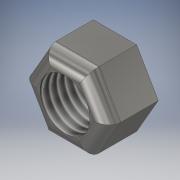
# Autodesk Inventor part: LucasCharles part 5 nut final
Saved by Autodesk Inventor 2018 (Build 220112000, 112)
## iProperties
Created: 2018-05-16
Part Number: LucasCharles part 5 nut final
Material: Stainless Steel, Austenitic
Document SubType Name: Modeling
Designer: 21lsilva
Density: 8 g/cm^3
Appearance: Semi-Polished
Author: 21lsilva
Autodesk Inventor part; units mm, degrees
ref_plane "YZ Plane" through (0, 0, 0) normal (1, 0, 0) x (0, 1, 0)
ref_plane "XZ Plane" through (0, 0, 0) normal (0, 1, 0) x (-1, 0, 0)
ref_plane "XY Plane" through (0, 0, 0) normal (0, 0, 1) x (1, 0, 0)
sketch "Sketch1" plane through (0, 0, 0) normal (0, 0, 1) x (1, 0, 0)
  line L0 (-10.9985, 0) -> (-5.4993, 9.525)
  line L1 (-5.4993, 9.525) -> (5.4993, 9.525)
  line L2 (5.4993, 9.525) -> (10.9985, 0)
  line L3 (10.9985, 0) -> (5.4993, -9.525)
  line L4 (5.4993, -9.525) -> (-5.4993, -9.525)
  line L5 (-5.4993, -9.525) -> (-10.9985, 0)
  point P0 (0, 0)
  point P1 (0, 0)
  dimension "d0" = 19.05
  constraints: 12 end point, 1 coincident, 13 other
  measures "d0" distance between parallel lines of L4 L1
extrude "Extrusion1" add sketch "Sketch1" along normal blind 12.7
sketch "Sketch2" plane through (0, 0, 12.7) normal (0, 0, 1) x (1, 0, 0)
  circle A0 centre (0, 0) radius 6.35
  dimension "d3" = 12.7
  constraints: 1 centre point, 1 coincident
  measures "d3" diameter of A0
extrude "Extrusion2" cut sketch "Sketch2" against normal blind 12.7
thread "Thread1" size "1/2-13 UNC" class "2B" standard "ANSI Unified Screw Threads" full length
fillet "Fillet1" radius 3.175 6 edges at (0, 9.525, 12.7) (8.2489, 4.7625, 12.7) (8.2489, -4.7625, 12.7) (0, -9.525, 12.7) (-8.2489, -4.7625, 12.7) (-8.2489, 4.7625, 12.7)
body "Solid1"
